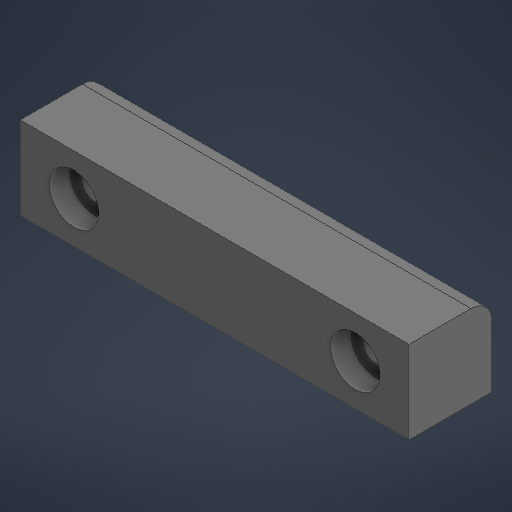
# Autodesk Inventor part: Satupofa
Saved by Autodesk Inventor 2025 (Build 290162010, 162A)
## iProperties
Created: 2025-02-13
Part Number: Satupofa
Material: Generic
Document SubType Name: Modeling
Designer: petruska.milan
Density: 1 g/cm^3
Appearance: Default
Author: petruska.milan
Autodesk Inventor part; units mm, degrees
ref_plane "YZ Plane" through (0, 0, 0) normal (1, 0, 0) x (0, 1, 0)
ref_plane "XZ Plane" through (0, 0, 0) normal (0, 1, 0) x (-1, 0, 0)
ref_plane "XY Plane" through (0, 0, 0) normal (0, 0, 1) x (1, 0, 0)
sketch "Sketch1" plane through (0, 0, 0) normal (0, 0, 1) x (1, 0, 0)
  line L0 (-23.5, -5) -> (23.5, -5)
  line L1 (23.5, -5) -> (23.5, 5)
  line L2 (23.5, 5) -> (-23.5, 5)
  line L3 (-23.5, 5) -> (-23.5, -5)
  line L4 (-23.5, -5) -> (23.5, 5) construction
  line L5 (23.5, -5) -> (-23.5, 5) construction
  point P0 (0, 0)
  dimension "d0" = 47
  dimension "d1" = 10
  constraints: 12 end point, 2 midpoint, 2 parallel, 1 horizontal, 1 perpendicular
  measures "d0" distance of L2.end L1.end
  measures "d1" distance of L1.end L0.end
extrude "Extrusion1" add sketch "Sketch1" along normal blind 10
sketch "Sketch2" plane through (0, 0, 10) normal (0, 0, 1) x (1, 0, 0)
  line L0 (-23.5, 5) -> (-23.5, -5) projected
  line L1 (-23.5, 0) -> (-17, 0)
  line L2 (-17, 0) -> (17, 0)
  point P0 (0, 0)
  dimension "d4" = 6.5
  dimension "d5" = 34
  constraints: 4 end point, 2 coincident, 1 horizontal, 1 midpoint, 1 point on line
  measures "d4" distance of L1.start L1.end
  measures "d5" distance of L1.end L2.end
hole "Hole1" at (-17, 0, 10) at (17, 0, 10) direction (0, 0, -1) diameter 3.2 end through all counterbore diameter 6 counterbore depth 2.5
fillet "Fillet1" radius 2.5 1 edges at (0, 5, 0)
body "Solid1"
